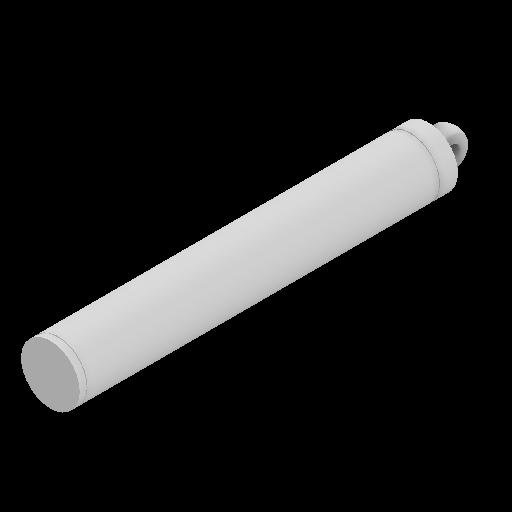
# Autodesk Inventor part: 1610-50H-2KG-12V-B07-Body
Saved by Autodesk Inventor 2025.2 (Build 292293000, 293)
## iProperties
Created: 2026-01-24
Part Number: 1610-50H-2KG-12V-B07-Body
Material: Generic
Document SubType Name: Modeling
Designer: valer
Density: 1 g/cm^3
Appearance: Default
Author: valer
Autodesk Inventor part; units mm, degrees
ref_plane "YZ Plane" through (0, 0, 0) normal (1, 0, 0) x (0, 1, 0)
ref_plane "XZ Plane" through (0, 0, 0) normal (0, 1, 0) x (-1, 0, 0)
ref_plane "XY Plane" through (0, 0, 0) normal (0, 0, 1) x (1, 0, 0)
sketch "Base" plane through (0, 0, 0) normal (0, 0, 1) x (1, 0, 0)
  circle A0 centre (0, 0) radius 8
  dimension "d0" = 16
  constraints: 1 centre point, 1 coincident
  measures "d0" diameter of A0
extrude "BaseFeature" add sketch "Base" along normal blind 5
sketch "Mount" plane through (0, 0, 0) normal (0, 0, -1) x (-1, 0, 0)
  line L0 (2.5, -5) -> (-2.5, -5)
  line L1 (-2.5, -5) -> (-2.5, 5)
  line L2 (-2.5, 5) -> (2.5, 5)
  line L3 (2.5, 5) -> (2.5, -5)
  line L4 (11.2, 0) -> (-11.2, 0) construction
  line L5 (0, -11.2) -> (0, 11.2) construction
  circle A0 centre (0, 0) radius 5
  point P0 (0, -5)
  point P1 (2.5, 4.3301)
  point P2 (-2.5, 4.3301)
  point P3 (-2.5, -4.3301)
  point P4 (2.5, -4.3301)
  dimension "d3" = 10
  dimension "d4" = 5
  constraints: 8 end point, 2 parallel, 2 tangent, 1 centre point, 1 coincident, 1 horizontal, 1 midpoint, 1 perpendicular, 1 point on line
  measures "d3" diameter of A0
  measures "d4" distance of L0.start L0.end
extrude "MountFeature" add sketch "Mount" along normal blind 9 contours A0 L1 L3
sketch "MountProfile" plane through (0, 0, 0) normal (1, 0, 0) x (0, 1, 0)
  line L0 (5, 0) -> (5, -9) projected
  line L1 (4.3301, -9) -> (5, -9) projected
  line L2 (4.3301, -9) -> (-4.3301, -9) projected
  line L3 (-5, -9) -> (-4.3301, -9) projected
  line L4 (-5, 0) -> (-5, -9) projected
  line L5 (8, 0) -> (-8, 0) projected
  circle A0 centre (0, -4) radius 5
  line L6 (5, -4) -> (-5, -4)
  line L7 (0, -11.8) -> (0, 7.8) projected
  point P0 (0, 0)
  point P1 (0, -4)
  point P2 (0, -9)
  point P3 (-5, -4)
  point P4 (5, -4)
  constraints: 3 tangent, 2 end point, 2 point on line, 1 centre point, 1 coincident, 1 midpoint, 1 perpendicular
revolve "MountProfileFeature" cut sketch "MountProfile" angle 360 about axis through (0, 0, -10) along (0, 0, 1) contours L0 L1 L2 A0 | L2 L3 L4 A0
sketch "MountHole" plane through (2.5, -4.3301, 0) normal (1, 0, 0) x (0, 0, -1)
  arc A0 (4, 0) -> (4, 8.6603) centre (4, 4.3301) ccw projected
  circle A1 centre (4, 4.3301) radius 2
  point P0 (0, 4.3301)
  dimension "d15" = 4
  constraints: 1 centre point, 1 coincident
  measures "d15" diameter of A1
extrude "MountHoleFeature" cut sketch "MountHole" against normal blind 10
sketch "Body" plane through (0, 0, 5) normal (0, 0, 1) x (1, 0, 0)
  circle A0 centre (0, 0) radius 8 projected
extrude "BodyFeature" add sketch "Body" along normal blind 96
ref_plane "BodyCapPlane" through (0, 0, 101) normal (0, 0, 1) x (1, 0, 0)
ref_plane "BaseBodyPlane" through (0, 0, 5) normal (0, 0, 1) x (1, 0, 0)
sketch "Sketch9" plane through (0, 0, 101) normal (0, 0, 1) x (1, 0, 0)
  circle A0 centre (0, 0) radius 8 projected
extrude "BodyCapFeature" add sketch "Sketch9" along normal blind 2
sketch "BodyCapEtch" plane through (0, 0, 101) normal (0, 0, 1) x (1, 0, 0)
  circle A0 centre (0, 0) radius 8 projected
  circle A1 centre (0, 0) radius 7.75
  dimension "d24" = 0.25
  constraints: 1 centre point, 1 coincident
  measures "d24" radial gap between concentric circles of A0 A1
extrude "BodyCapEtchFeature" cut sketch "BodyCapEtch" along normal mid plane 0.25
sketch "BodyBaseEtch" plane through (0, 0, 5) normal (0, 0, 1) x (1, 0, 0)
  circle A0 centre (0, 0) radius 8 projected
  circle A1 centre (0, 0) radius 7.75
  dimension "d27" = 0.25
  constraints: 1 centre point, 1 coincident
  measures "d27" radial gap between concentric circles of A0 A1
extrude "BodyBaseEtchFeature" cut sketch "BodyBaseEtch" along normal mid plane 0.25
body "Solid1"
